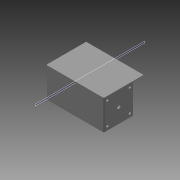
# Autodesk Inventor part: base
Saved by Autodesk Inventor 2015 (Build 190159000, 159)
## iProperties
Created: 2015-02-18
Part Number: base
Material: Genérico
Document SubType Name: Modeling
Designer: jorge
Density: 1 g/cm^3
Appearance: Valor por defecto
Author: jorge
Autodesk Inventor part; units mm, degrees
note: some values were not read from the file. Chosen so that the rebuilt part matches the saved one: direction of "Agujero1"; direction of "Agujero2"; direction of "Agujero3".
ref_plane "YZ Plane" through (0, 0, 0) normal (1, 0, 0) x (0, 1, 0)
ref_plane "XZ Plane" through (0, 0, 0) normal (0, 1, 0) x (-1, 0, 0)
ref_plane "XY Plane" through (0, 0, 0) normal (0, 0, 1) x (1, 0, 0)
sketch "Boceto1" plane through (0, 0, 0) normal (0, 0, 1) x (1, 0, 0)
  line L0 (105, 0) -> (105, 24.5) projected
  line L1 (0, 24.5) -> (0, 0) projected
  line L2 (105, 24.5) -> (0, 24.5)
  line L3 (113, 129.5) -> (-8, 129.5)
  line L4 (-8, 129.5) -> (-8, -80.5)
  line L5 (-8, -80.5) -> (113, -80.5)
  line L6 (113, -80.5) -> (113, 129.5)
  line L7 (113, 129.5) -> (-8, -80.5) construction
  line L8 (-8, 129.5) -> (113, -80.5) construction
  point P0 (52.5, 24.5)
  dimension "d0" = 121
  dimension "d1" = 210
  constraints: 14 end point, 3 midpoint, 2 horizontal, 2 parallel, 1 perpendicular
  measures "d0" distance of L5.end L4.end
  measures "d1" distance of L4.end L3.end
extrude "Extrusión1" add sketch "Boceto1" along normal blind 3
sketch "Boceto2" plane through (0, 0, 0) normal (0, 0, -1) x (-1, 0, 0)
  line L0 (0, 53) -> (5, 53) projected
  line L1 (0, -4) -> (5, -4) projected
  line L2 (5, 53) -> (8, 53)
  line L3 (8, 129.5) -> (8, -80.5) projected
  line L4 (5, -4) -> (8, -4)
  line L5 (8, -4) -> (8, 53)
  line L6 (8, 53) -> (5, 53)
  line L7 (5, 53) -> (5, -4)
  point P0 (0, 0)
  constraints: 10 end point, 2 horizontal, 2 parallel, 1 perpendicular, 1 point on line
ref_plane "Plano de trabajo1" through (52.5, -80.5, 0) normal (-1, 0, 0) x (0, 0, 1)
extrude "Extrusión2" add sketch "Boceto2" along normal blind 60
sketch "Boceto3" plane through (-8, -80.5, 3) normal (-1, 0, 0) x (0, 0, 1)
  circle A0 centre (-54.9977, 81.5) radius 3 projected
  circle A1 centre (-54.9977, 128.5) radius 3 projected
  circle A2 centre (-7.9977, 128.5) radius 3 projected
  circle A3 centre (-7.9977, 81.5) radius 3 projected
  point P0 (-3, 80.5)
hole "Agujero1" at (-8, 1, -51.9977) at (-8, 48, -51.9977) at (-8, 48, -4.9977) at (-8, 1, -4.9977) direction (1, 0, 0) diameter 5 end up to surface
sketch "Boceto4" plane through (-8, -80.5, 3) normal (-1, 0, 0) x (0, 0, 1)
  circle A0 centre (-31.4977, 105) radius 4 projected
  circle A1 centre (-31.4977, 105) radius 4
  point P0 (-3, 80.5)
  dimension "d13" = 8
  constraints: 1 centre point, 1 coincident
  measures "d13" diameter of A1
hole "Agujero2" at (-8, 24.5, -28.4977) direction (1, 0, 0) diameter 8 end up to surface
sketch "Boceto5" plane through (-8, 53, 0) normal (0, 1, 0) x (1, 0, 0)
  line L0 (3, 0) -> (33, 0)
  line L1 (33, 0) -> (33, 60)
  line L2 (33, 60) -> (3, 60)
  line L3 (3, 60) -> (0, 60)
  line L4 (0, 60) -> (0, 0)
  line L5 (0, 0) -> (3, 0)
  line L6 (33, 60) -> (33, 0)
  line L7 (33, 60) -> (0, 60)
  line L8 (0, 60) -> (0, 0)
  line L9 (0, 0) -> (33, 0)
  line L10 (33, 0) -> (33, 60)
  point P0 (8, 0)
  dimension "d21" = 30
  dimension "d22" = 60
  constraints: 22 end point, 4 perpendicular, 3 parallel, 2 horizontal, 1 vertical
  measures "d21" distance of L2.end L1.end
  measures "d22" distance of L1.end L0.end
extrude "Extrusión3" add sketch "Boceto5" along normal blind 3
sketch "Boceto6" plane through (-8, 56, 0) normal (0, 1, 0) x (1, 0, 0)
  circle A0 centre (8.88, 50.6734) radius 0.889 projected
  circle A1 centre (24.12, 50.6734) radius 0.889 projected
  circle A2 centre (24.12, 10.0334) radius 0.889 projected
  circle A3 centre (8.88, 10.0334) radius 0.889 projected
  point P0 (8, 0)
hole "Agujero3" at (16.12, 56, -50.6734) at (0.88, 56, -50.6734) at (16.12, 56, -10.0334) at (0.88, 56, -10.0334) direction (0, -1, 0) diameter 2 end up to surface
mirror "Simetría1" about plane through (52.5, -80.5, 0) normal (-1, 0, 0) of "Extrusión3", "Agujero2", "Agujero1", "Extrusión2"
fillet "Empalme1" radius 2 2 edges at (96.5, 56, 0) (8.5, 56, 0)
sketch "Boceto7" plane through (0, 0, 0) normal (0, 0, -1) x (-1, 0, 0)
  line L0 (8, -4) -> (8, -7)
  line L1 (8, -4) -> (8, -80.5) projected
  line L2 (8, -7) -> (-113, -7)
  line L3 (-113, -80.5) -> (-113, 129.5) projected
  line L4 (-113, -80.5) -> (-113, -7)
  line L5 (-113, -80.5) -> (-113, -4) projected
  line L6 (-113, -80.5) -> (8, -80.5)
  line L7 (8, -80.5) -> (8, -7)
  point P0 (0, 0)
  dimension "d33" = 3
  constraints: 10 end point, 2 collinear, 2 point on line, 1 horizontal, 1 perpendicular
  measures "d33" distance of L0.start L0.end
extrude "Extrusión4" cut sketch "Boceto7" against normal blind 3
sketch "Boceto8" plane through (0, 0, 0) normal (0, 0, -1) x (-1, 0, 0)
  line L0 (-113, -4) -> (-113, -7)
  line L1 (-113, -7) -> (8, -7)
  line L2 (8, -7) -> (8, -4)
  line L3 (8, -4) -> (-113, -4)
  point P0 (0, 0)
  dimension "d36" = 3
  dimension "d37" = 121
  dimension "d38" = 3
  constraints: 8 end point, 2 perpendicular, 1 vertical
  measures "d36" distance of L0.start L0.end
  measures "d37" distance of L0.end L1.end
  measures "d38" distance of L1.end L2.end
extrude "Extrusión5" add sketch "Boceto8" along normal blind 60
sketch "Boceto9" plane through (0, 0, -60) normal (0, 0, -1) x (-1, 0, 0)
  point P0 (0, 0)
sketch "Boceto10" plane through (0, 0, 0) normal (0, 0, -1) x (-1, 0, 0)
  line L0 (-46.8669, 72) -> (-100.1331, 72) projected
  line L1 (-46.8669, 77) -> (-100.1331, 77)
  line L2 (-100.1331, 77) -> (-113, 77)
  line L3 (-113, 58) -> (-113, 129.5) projected
  line L4 (-46.8669, 77) -> (6.9064, 77)
  line L5 (6.9064, 77) -> (8, 77)
  line L6 (8, 129.5) -> (8, 58) projected
  line L7 (-113, 77) -> (8.9757, 77)
  line L8 (8.9757, 77) -> (8.9757, 129.5)
  line L9 (8.9757, 129.5) -> (-113, 129.5)
  line L10 (-113, 129.5) -> (-113, 77)
  point P0 (0, 0)
  dimension "d41" = 5
  constraints: 16 end point, 3 horizontal, 3 parallel, 3 point on line, 1 perpendicular
  measures "d41" distance between parallel lines of L0 L1
extrude "Extrusión6" cut sketch "Boceto10" against normal blind 10
fillet "Empalme2" radius 2 11 edges at (-5, 53, -30) (-8, 56.5858, -0.5858) (-8, 67.5, 0) (-8, 56, -31) (-5, -4, -30) (110, -4, -30) (110, 53, -30) (113, 56.5858, -0.5858) (113, 67.5, 0) (113, 56, -31) (52.5, 77, 0)
fillet "Empalme3" radius 2 2 edges at (80, 53, -30) (25, 53, -30)
fillet "Empalme4" radius 2 2 edges at (113, -7, -28.5) (-8, -7, -28.5)
